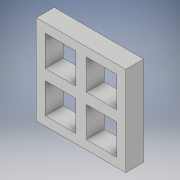
# Autodesk Inventor part: Hydrogel_Test
Saved by Autodesk Inventor 2018 (Build 220112000, 112)
## iProperties
Created: 2020-01-23
Part Number: Hydrogel_Test
Material: Generisch
Document SubType Name: Modeling
Designer: maxse
Density: 1 g/cm^3
Appearance: Vorgabe
Author: maxse
Autodesk Inventor part; units mm, degrees
ref_plane "YZ Plane" through (0, 0, 0) normal (1, 0, 0) x (0, 1, 0)
ref_plane "XZ Plane" through (0, 0, 0) normal (0, 1, 0) x (-1, 0, 0)
ref_plane "XY Plane" through (0, 0, 0) normal (0, 0, 1) x (1, 0, 0)
sketch "Skizze1" plane through (0, 0, 0) normal (0, 1, 0) x (-1, 0, 0)
  line L0 (-12.5, 12.5) -> (12.5, 12.5)
  line L1 (12.5, 12.5) -> (12.5, -12.5)
  line L2 (12.5, -12.5) -> (-12.5, -12.5)
  line L3 (-12.5, -12.5) -> (-12.5, 12.5)
  line L4 (-12.5, 12.5) -> (12.5, -12.5) construction
  line L5 (12.5, 12.5) -> (-12.5, -12.5) construction
  line L6 (10, 10) -> (1.5, 10)
  line L7 (1.5, 10) -> (1.5, 1.5)
  line L8 (1.5, 1.5) -> (10, 1.5)
  line L9 (10, 1.5) -> (10, 10)
  line L10 (10, -10) -> (1.5, -10)
  line L11 (1.5, -10) -> (1.5, -1.5)
  line L12 (1.5, -1.5) -> (10, -1.5)
  line L13 (10, -1.5) -> (10, -10)
  line L14 (-1.5, 1.5) -> (-10, 1.5)
  line L15 (-10, 1.5) -> (-10, 10)
  line L16 (-10, 10) -> (-1.5, 10)
  line L17 (-1.5, 10) -> (-1.5, 1.5)
  line L18 (-1.5, -1.5) -> (-10, -1.5)
  line L19 (-10, -1.5) -> (-10, -10)
  line L20 (-10, -10) -> (-1.5, -10)
  line L21 (-1.5, -10) -> (-1.5, -1.5)
  point P0 (0, 0)
  dimension "d0" = 25
  dimension "d1" = 25
  dimension "d2" = 8.5
  dimension "d3" = 8.5
  dimension "d4" = 8.5
  dimension "d5" = 8.5
  dimension "d6" = 8.5
  dimension "d7" = 8.5
  dimension "d8" = 8.5
  dimension "d9" = 8.5
  dimension "d10" = 2.5
  dimension "d11" = 2.5
  dimension "d12" = 2.5
  constraints: 44 end point, 10 parallel, 5 horizontal, 5 perpendicular, 5 point on line, 2 midpoint
  measures "d0" distance of L1.end L2.end
  measures "d1" distance of L0.end L1.end
  measures "d2" distance of L8.end L7.end
  measures "d3" distance of L7.end L6.end
  measures "d4" distance of L11.end L12.end
  measures "d5" distance of L10.end L11.end
  measures "d6" distance of L15.end L16.end
  measures "d7" distance of L14.end L15.end
  measures "d8" distance of L20.end L19.end
  measures "d9" distance of L19.end L18.end
  measures "d10" distance between parallel lines of L1 L9
  measures "d11" distance between parallel lines of L2 L10
  measures "d12" distance between parallel lines of L3 L15
extrude "Extrusion1" add sketch "Skizze1" along normal blind 5
